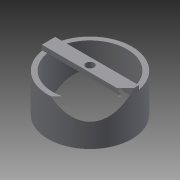
# Autodesk Inventor part: tunnel
Saved by Autodesk Inventor 2014 SP2 (Build 180246200, 246)
## iProperties
Created: 2016-03-11
Part Number: tunnel
Material: Generic
Document SubType Name: Modeling
Designer: schrluka
Density: 1 g/cm^3
Appearance: Default
Author: schrluka
Autodesk Inventor part; units mm, degrees
ref_plane "YZ Plane" through (0, 0, 0) normal (1, 0, 0) x (0, 1, 0)
ref_plane "XZ Plane" through (0, 0, 0) normal (0, 1, 0) x (-1, 0, 0)
ref_plane "XY Plane" through (0, 0, 0) normal (0, 0, 1) x (1, 0, 0)
sketch "Sketch1" plane through (0, 0, 0) normal (0, 0, 1) x (1, 0, 0)
  spline S0 degree 3 poles (-37.25, 0) (-37.25, -7.0376) (-35.2039, -14.0633) (-31.4252, -20.0004) (-27.6466, -25.9375) (-22.1482, -30.766) (-15.7726, -33.7459) (-9.397, -36.7258) (-2.1659, -37.8471) (4.8127, -36.9378) (11.7914, -36.0285) (18.4938, -33.0918) (23.893, -28.5778) (29.2921, -24.0637) (33.3697, -17.9875) (35.5009, -11.2804) (37.6321, -4.5732) (37.8097, 2.7422) (36.0064, 9.5448) (34.2031, 16.3475) (30.4251, 22.6143) (25.2512, 27.385) (20.0774, 32.1557) (13.5254, 35.414) (6.5991, 36.6608) (-0.3272, 37.9076) (-7.6042, 37.1385) (-14.1169, 34.4714) (-20.6295, 31.8043) (-26.3557, 27.2483) (-30.4179, 21.5014) (-34.4802, 15.7546) (-36.8647, 8.8365) (-37.2061, 1.8072) (-37.2354, 1.2052) (-37.25, 0.6026) (-37.25, 0) knots 0 0 0 0 0.566787 0.566787 0.566787 1.133573 1.133573 1.133573 1.70036 1.70036 1.70036 2.267146 2.267146 2.267146 2.833933 2.833933 2.833933 3.400719 3.400719 3.400719 3.967506 3.967506 3.967506 4.534292 4.534292 4.534292 5.101079 5.101079 5.101079 5.667865 5.667865 5.667865 6.234652 6.234652 6.234652 6.283185 6.283185 6.283185 6.283185 projected
  spline S1 degree 5 poles (-38.75, 0) (-38.7501, -2.7047) (-38.5078, -5.4094) (-38.0316, -8.0852) (-36.6239, -13.33) (-34.3392, -18.2559) (-32.9845, -20.6148) (-29.8595, -25.0561) (-26.0175, -28.8925) (-23.9357, -30.6396) (-19.4934, -33.7614) (-14.5735, -36.0618) (-12.0149, -36.9831) (-6.7678, -38.3822) (-1.3581, -38.8593) (1.3604, -38.8675) (6.7714, -38.3973) (12.0133, -36.9798) (14.5666, -36.049) (19.4877, -33.7543) (23.9437, -30.6512) (26.0275, -28.9023) (29.8573, -25.0529) (32.972, -20.6052) (34.3321, -18.2523) (36.6385, -13.3362) (38.0403, -8.0889) (38.5046, -5.4103) (38.9743, 0) (38.5079, 5.4103) (38.0448, 8.0901) (36.6331, 13.3345) (34.3305, 18.2516) (32.9714, 20.6051) (29.8608, 25.0551) (26.0293, 28.9037) (23.9413, 30.647) (19.4872, 33.7528) (14.5665, 36.0499) (12.0141, 36.984) (6.7708, 38.3997) (1.3596, 38.8619) (-1.3583, 38.8577) (-6.7678, 38.3823) (-12.0157, 36.988) (-14.5739, 36.063) (-19.4902, 33.7565) (-23.9357, 30.6394) (-26.0178, 28.8927) (-29.8639, 25.0602) (-32.9831, 20.614) (-34.3346, 18.2543) (-36.6237, 13.3303) (-38.0331, 8.0858) (-38.5138, 5.4104) (-38.7506, 2.7047) (-38.75, 0) knots 0 0 0 0 0 0 0.055551 0.055551 0.055551 0.111119 0.111119 0.111119 0.166658 0.166658 0.166658 0.222223 0.222223 0.222223 0.277783 0.277783 0.277783 0.333326 0.333326 0.333326 0.388895 0.388895 0.388895 0.444438 0.444438 0.444438 0.499998 0.499998 0.499998 0.555563 0.555563 0.555563 0.611102 0.611102 0.611102 0.66667 0.66667 0.66667 0.722222 0.722222 0.722222 0.777772 0.777772 0.777772 0.83334 0.83334 0.83334 0.88888 0.88888 0.88888 0.944445 0.944445 0.944445 1 1 1 1 1 1
  spline S2 degree 5 poles (-43.75, 0) (-43.7501, -3.0529) (-43.4775, -6.1058) (-42.9407, -9.1264) (-41.3515, -15.0495) (-38.7703, -20.6121) (-37.2389, -23.2767) (-33.7116, -28.2913) (-29.3743, -32.6225) (-27.0258, -34.5933) (-22.0107, -38.1167) (-16.4569, -40.7135) (-13.5672, -41.7555) (-7.641, -43.3364) (-1.5309, -43.8747) (1.5391, -43.8827) (7.6467, -43.3509) (13.5639, -41.7524) (16.4449, -40.7023) (22.0015, -38.1117) (27.0322, -34.6069) (29.3867, -32.6308) (33.7119, -28.2852) (37.2284, -23.263) (38.763, -20.6081) (41.3648, -15.0583) (42.9484, -9.1357) (43.4738, -6.1111) (44.0049, -0.0005) (43.4774, 6.1102) (42.9529, 9.1371) (41.3593, 15.0572) (38.7607, 20.6082) (37.2277, 23.2632) (33.7158, 28.2869) (29.3897, 32.6312) (27.0312, 34.6016) (22.0016, 38.1099) (16.4443, 40.7036) (13.5628, 41.7573) (7.6441, 43.3536) (1.5365, 43.877) (-1.5313, 43.873) (-7.6403, 43.3367) (-13.5665, 41.7609) (-16.4565, 40.7151) (-22.0073, 38.1119) (-27.0262, 34.5928) (-29.3749, 32.6223) (-33.7159, 28.2954) (-37.237, 23.2766) (-38.7649, 20.6118) (-41.3507, 15.0514) (-42.9418, 9.1288) (-43.4834, 6.1081) (-43.7506, 3.0536) (-43.75, 0) knots 0 0 0 0 0 0 0.055537 0.055537 0.055537 0.111144 0.111144 0.111144 0.166635 0.166635 0.166635 0.222228 0.222228 0.222228 0.277799 0.277799 0.277799 0.333305 0.333305 0.333305 0.388916 0.388916 0.388916 0.444424 0.444424 0.444424 0.499992 0.499992 0.499992 0.555587 0.555587 0.555587 0.611077 0.611077 0.611077 0.666684 0.666684 0.666684 0.722224 0.722224 0.722224 0.777757 0.777757 0.777757 0.833365 0.833365 0.833365 0.888857 0.888857 0.888857 0.944449 0.944449 0.944449 1 1 1 1 1 1
  point P0 (0, 0)
  point P1 (-37.25, 0)
  dimension "d0" = 1.5
  dimension "d1" = 6.5
  constraints: 4 other
extrude "Extrusion1" add sketch "Sketch1" against normal blind 40 contours S2
sketch "Sketch5" plane through (0, 0, 0) normal (0, 0, 1) x (1, 0, 0)
  line L0 (-43.75, -6.6095) -> (43.7402, -6.6095)
  line L1 (43.7402, -6.6095) -> (43.7402, 7.3905)
  line L2 (43.7402, 7.3905) -> (-43.75, 7.3905)
  line L3 (-43.75, 7.3905) -> (-43.75, -6.6095)
  line L4 (-43.75, -6.6095) -> (43.7402, 7.3905) construction
  line L5 (43.7402, -6.6095) -> (-43.75, 7.3905) construction
  point P0 (-38.75, 0)
  point P1 (-0.0049, 0.3905)
  dimension "d27" = 14
  constraints: 12 end point, 2 midpoint, 2 parallel, 2 vertical, 1 horizontal, 1 perpendicular, 1 other
  measures "d27" distance of L2.end L0.start
extrude "Extrusion5" add sketch "Sketch5" along normal blind 5
sketch "Sketch6" plane through (0, 0, 5) normal (0, 0, 1) x (1, 0, 0)
  point P0 (0, 0)
  point P1 (0, 0)
  constraints: 1 coincident
hole "Hole1" at (0, 0, 5) direction (0, 0, -1) diameter 8.5 end through all
body "Solid1"
